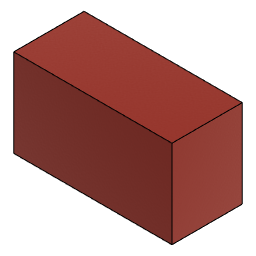
锂电池20x25x45mm v1 (Autodesk Fusion 360 design; units mm, degrees)
Autodesk Fusion 360 part; units mm, degrees
sketch "草图1" plane through (0, 0, 0) normal (0, 0, 1) x (1, 0, 0)
  line L0 (-33.7684, 16.7793) -> (11.2316, 16.7793)
  line L1 (11.2316, 16.7793) -> (11.2316, -3.2207)
  line L2 (11.2316, -3.2207) -> (-33.7684, -3.2207)
  line L3 (-33.7684, -3.2207) -> (-33.7684, 16.7793)
  dimension "d1" = 45
  dimension "d2" = 20
  constraint horizontal L0
  constraint vertical L1
  constraint horizontal L2
  constraint vertical L3
  measures "d1" distance of L0.start L0.end
  measures "d2" distance of L0.start L2.end
extrude "拉伸1" add sketch "草图1" along normal blind 25
